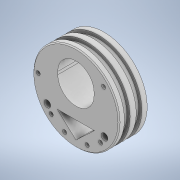
# Autodesk Inventor part: CameraFrontSupport
Saved by Autodesk Inventor 2020 (Build 240168000, 168)
## iProperties
Created: 2019-08-28
Part Number: CameraFrontSupport
Material: Generic
Document SubType Name: Modeling
Designer: rosbo
Density: 1 g/cm^3
Appearance: Default
Author: rosbo
Autodesk Inventor part; units mm, degrees
sketch "Sketch1" plane through (0, 0, 0) normal (0, 0, 1) x (1, 0, 0)
  circle A0 centre (0, 0) radius 37.7444
  dimension "d0" = 75.4888
  constraints: 1 centre point, 1 coincident
  measures "d0" diameter of A0
extrude "Extrusion1" add sketch "Sketch1" along normal blind 27.94
ref_plane "Work Plane1" through (0, 0, 21.59) normal (0, 0, 1) x (1, 0, 0)
sketch "Sketch2" plane through (0, 0, 21.59) normal (0, 0, 1) x (1, 0, 0)
  circle A0 centre (0, 0) radius 34.9504
  circle A1 centre (0, 0) radius 37.7444 projected
  dimension "d4" = 2.794
  constraints: 1 centre point, 1 coincident
  measures "d4" radial gap between concentric circles of A0 A1
extrude "Extrusion2" cut sketch "Sketch2" against normal blind 4.953
ref_plane "Work Plane2" through (0, 0, 6.35) normal (0, 0, -1) x (-1, 0, 0)
sketch "Sketch3" plane through (0, 0, 6.35) normal (0, 0, -1) x (-1, 0, 0)
  circle A0 centre (0, 0) radius 34.9504
  circle A1 centre (0, 0) radius 37.7444 projected
  dimension "d8" = 2.794
  constraints: 1 centre point, 1 coincident
  measures "d8" radial gap between concentric circles of A0 A1
extrude "Extrusion3" cut sketch "Sketch3" against normal blind 4.953
sketch "Sketch4" plane through (0, 0, 0) normal (0, 0, -1) x (-1, 0, 0)
  circle A0 centre (0, 0) radius 31.7754
  line L0 (-29.1271, -12.7) -> (29.1271, -12.7)
  line L1 (-19.685, -12.7) -> (-19.685, 24.9435)
  line L2 (19.685, -12.7) -> (19.685, 24.9435)
  line L3 (0, -52.8422) -> (0, 52.8422) projected
  circle A1 centre (0, 0) radius 37.7444 projected
  line L4 (52.8422, 0) -> (-52.8422, 0) projected
  dimension "d11" = 39.37
  dimension "d12" = 5.969
  dimension "d25" = 12.7
  constraints: 6 end point, 4 point on circle, 2 point on line, 1 centre point, 1 coincident, 1 horizontal, 1 perpendicular, 1 vertical, 1 other
  measures "d11" distance between parallel lines of L2 L1
  measures "d12" radial gap between concentric circles of A1 A0
  measures "d25" distance between parallel lines of L4 L0
extrude "Extrusion4" [suppressed]
sketch "Sketch5" plane through (0, 0, 27.94) normal (0, 0, 1) x (1, 0, 0)
  circle A0 centre (24.257, 20.828) radius 1.778
  circle A1 centre (-21.59, -22.86) radius 1.778
  circle A2 centre (21.59, -22.86) radius 1.778
  line L0 (0, -52.8422) -> (0, 52.8422) projected
  line L1 (-52.8422, 0) -> (52.8422, 0) projected
  circle A3 centre (-33.02, 2.54) radius 1.778
  point P0 (0, 0)
  dimension "d16" = 3.556
  dimension "d17" = 3.556
  dimension "d18" = 3.556
  dimension "d19" = 20.828
  dimension "d20" = 24.257
  dimension "d21" = 22.86
  dimension "d22" = 21.59
  dimension "d64" = 3.556
  dimension "d65" = 2.54
  dimension "d66" = 33.02
  constraints: 4 centre point, 1 symmetric about line
  measures "d16" diameter of A0
  measures "d17" diameter of A1
  measures "d18" diameter of A2
  measures "d19" distance from line of A0.centre L1
  measures "d20" distance from line of L0 A0.centre
  measures "d21" vertical distance of point (0, 0) A2.centre
  measures "d22" distance from line of A2.centre L0
  measures "d64" diameter of A3
  measures "d65" distance from line of L1 A3.centre
  measures "d66" distance from line of L0 A3.centre
extrude "Extrusion5" cut sketch "Sketch5" against normal through all
sketch "Sketch6" plane through (0, 0, 27.94) normal (0, 0, 1) x (1, 0, 0)
  circle A0 centre (21.59, -22.86) radius 1.778 projected
  circle A1 centre (24.257, 20.828) radius 1.778 projected
  circle A2 centre (-21.59, -22.86) radius 1.778 projected
  circle A3 centre (0, 0) radius 37.7444 projected
  circle A4 centre (-21.59, -22.86) radius 1.778 projected
  circle A5 centre (-21.59, -22.86) radius 8.255
  circle A6 centre (21.59, -22.86) radius 8.255
  line L0 (-16.3153, -16.51) -> (26.8647, -16.51)
  circle A7 centre (0, 0) radius 34.9504 projected
  circle A8 centre (0, 0) radius 31.7754
  line L1 (0, -31.7754) -> (-16.2938, -16.51)
  line L2 (0, -31.7754) -> (16.2938, -16.51)
  dimension "d26" = 16.51
  dimension "d27" = 16.51
  constraints: 6 end point, 3 coincident, 2 point on line, 1 vertical alignment, 10 other
extrude "Extrusion6" cut sketch "Sketch6" against normal through all contours L2 L1 L0
fillet "Fillet1" [suppressed]
chamfer "Chamfer1" distance 2.54 angle 45 1 edges at (-37.7444, 0, 27.94)
sketch "Sketch9" plane through (0, 0, 27.94) normal (0, 0, 1) x (1, 0, 0)
  circle A0 centre (-9.8806, -30.607) radius 1.778
  circle A1 centre (9.8806, -30.607) radius 1.778
  line L0 (-52.8422, 0) -> (52.8422, 0) projected
  line L1 (0, -52.8422) -> (0, 52.8422) projected
  line L2 (-14.9225, -28.448) -> (14.9225, -28.448)
  line L3 (14.9225, -28.448) -> (14.9225, -34.163)
  line L4 (14.9225, -34.163) -> (-14.9225, -34.163)
  line L5 (-14.9225, -34.163) -> (-14.9225, -28.448)
  point P0 (0, 0)
  dimension "d45" = 3.556
  dimension "d46" = 3.556
  dimension "d47" = 19.7612
  dimension "d48" = 29.845
  dimension "d49" = 5.715
  dimension "d50" = 3.556
  dimension "d51" = 34.163
  constraints: 8 end point, 2 centre point, 2 parallel, 1 horizontal, 1 perpendicular, 1 symmetric about line, 1 other
  measures "d45" diameter of A1
  measures "d46" diameter of A0
  measures "d47" distance of A0.centre A1.centre
  measures "d48" distance between parallel lines of L3 L5
  measures "d49" distance between parallel lines of L2 L4
  measures "d50" distance from line of A1.centre L4
  measures "d51" distance between parallel lines of L4 L0
extrude "Extrusion9" cut sketch "Sketch9" against normal through all contours A0 | A1
sketch "Sketch11" plane through (0, 0, 0) normal (0, 0, -1) x (-1, 0, 0)
  circle A0 centre (-9.8806, -30.607) radius 1.778 projected
  circle A1 centre (9.8806, -30.607) radius 1.778 projected
  line L0 (16.2938, -16.51) -> (0, -31.7754) projected
  line L1 (0, -31.7754) -> (-16.2938, -16.51) projected
  line L2 (-16.2938, -16.51) -> (16.2938, -16.51) projected
  circle A2 centre (-21.59, -22.86) radius 1.778 projected
  circle A3 centre (-24.257, 20.828) radius 1.778 projected
  circle A4 centre (21.59, -22.86) radius 1.778 projected
  circle A5 centre (0, 0) radius 37.7444 projected
extrude "Extrusion10" cut sketch "Sketch11" against normal blind 1.651
sketch "Sketch12" plane through (0, 0, 27.94) normal (0, 0, 1) x (1, 0, 0)
  circle A0 centre (9.8806, -30.607) radius 1.778 projected
  circle A1 centre (-9.8806, -30.607) radius 1.778 projected
  circle A2 centre (-21.59, -22.86) radius 1.778 projected
  circle A3 centre (24.257, 20.828) radius 1.778 projected
  circle A4 centre (21.59, -22.86) radius 1.778 projected
  line L0 (0, -31.7754) -> (-16.2938, -16.51) projected
  line L1 (-16.2938, -16.51) -> (16.2938, -16.51) projected
  line L2 (16.2938, -16.51) -> (0, -31.7754) projected
  circle A5 centre (0, 0) radius 35.2044 projected
  circle A6 centre (0, 0) radius 37.7444 projected
extrude "Extrusion11" cut sketch "Sketch12" against normal blind 1.651 contours A0 | A1 | A2 | A3 | A4 | L0 L1 L2 | A5 | A6
ref_plane "Work Plane4" through (-16.2938, -35.56, 1.651) normal (0, -1, 0) x (1, 0, 0)
sketch "Sketch13" plane through (-16.2938, -35.56, 1.651) normal (0, -1, 0) x (1, 0, 0)
  line L0 (16.2938, -7.239) -> (16.2938, 31.877) projected
  line L1 (-36.5483, -1.651) -> (69.136, -1.651) projected
  line L2 (8.1912, 24.638) -> (8.1912, 0) projected
  line L3 (54.0382, 0) -> (-21.4506, 0) projected
  line L4 (-21.4506, 4.699) -> (54.0382, 4.699) projected
  line L5 (39.6618, 24.638) -> (39.6618, 0) projected
  line L6 (51.2442, 4.699) -> (-18.6566, 4.699) projected
  line L7 (-2.049, 0) -> (34.6366, 0) projected
  line L8 (13.1188, 4.699) -> (19.4688, 4.699)
  line L9 (19.4688, 4.699) -> (19.4688, 0)
  line L10 (19.4688, 0) -> (13.1188, 0)
  line L11 (13.1188, 0) -> (13.1188, 4.699)
  point P0 (16.2938, -1.651)
  point P1 (13.1188, 0)
  point P2 (19.4688, 0)
  dimension "d61" = 6.35
  constraints: 8 end point, 2 parallel, 2 point on line, 1 horizontal, 1 perpendicular, 1 other
  measures "d61" distance between parallel lines of L9 L11
extrude "Extrusion12" cut sketch "Sketch13" against normal mid plane 25.4 contours L3 L11 L4 L0 | L0 L4 L9 L3
sketch "Sketch14" plane through (0, 0, 1.651) normal (0, 0, -1) x (-1, 0, 0)
  circle A0 centre (-25.0506, -16.8477) radius 2.9591
  circle A1 centre (25.0506, -16.8477) radius 2.9591
  line L0 (52.8422, 0) -> (-52.8422, 0) projected
  line L1 (0, -52.8422) -> (0, 52.8422) projected
  arc A2 (3.175, -34.8059) -> (-3.175, -34.8059) centre (0, 0) ccw projected
  dimension "d67" = 5.9182
  dimension "d68" = 5.9182
  constraints: 2 centre point, 1 symmetric about line
  measures "d67" diameter of A0
  measures "d68" diameter of A1
extrude "Extrusion13" cut sketch "Sketch14" against normal through all contours A0 | A1
sketch "Sketch15" plane through (0, 0, 1.651) normal (0, 0, -1) x (-1, 0, 0)
  circle A0 centre (0, 11.0744) radius 15.875
  line L0 (0, 26.9494) -> (0, 37.7444)
  arc A1 (3.175, -37.6106) -> (-3.175, -37.6106) centre (0, 0) ccw projected
  dimension "d71" = 31.75
  dimension "d73" = 10.795
  constraints: 2 end point, 1 point on circle, 1 vertical, 1 vertical alignment, 2 other
  measures "d73" distance of L0.start L0.end
sketch "Sketch16" plane through (0, 0, 1.651) normal (0, 0, -1) x (-1, 0, 0)
  line L0 (0, 9.8044) -> (0, 12.3444) construction
  line L1 (15.875, 9.8044) -> (15.875, 12.3444)
  line L2 (-15.875, 12.3444) -> (-15.875, 9.8044)
  arc A0 (-15.875, 9.8044) -> (15.875, 9.8044) centre (0, 9.8044) ccw
  arc A1 (15.875, 12.3444) -> (-15.875, 12.3444) centre (0, 12.3444) ccw
  line L3 (0, -52.8422) -> (0, 52.8422) projected
  point P0 (0, 0)
  point P1 (0, 11.0744)
  dimension "d75" = 15.875
  dimension "d76" = 2.54
  constraints: 8 end point, 4 point on circle, 4 tangent, 2 centre point, 1 midpoint, 1 parallel, 1 point on line, 1 vertical
  measures "d75" radius of A1
  measures "d76" distance of L1.start L1.end
extrude "Extrusion14" cut sketch "Sketch16" against normal through all
body "Solid1"
